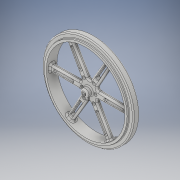
# Autodesk Inventor part: bepf_kolo_felga
Saved by Autodesk Inventor 2017 (Build 210142000, 142)
## iProperties
Created: 2016-11-22
Part Number: bepf_kolo_felga
Material: Tworzywo o ultrawysokiej masie cząsteczkowej, czarne
Document SubType Name: Modeling
Designer: gagato
Density: 0.94 g/cm^3
Appearance: Domyślna
Mass: 13.9753 g
Surface Area: 117.76 cm^2
Volume: 14.8674 cm^3
Author: gagato
Autodesk Inventor part; units mm, degrees
ref_plane "YZ Plane" through (0, 0, 0) normal (1, 0, 0) x (0, 1, 0)
ref_plane "XZ Plane" through (0, 0, 0) normal (0, 1, 0) x (-1, 0, 0)
ref_plane "XY Plane" through (0, 0, 0) normal (0, 0, 1) x (1, 0, 0)
sketch "Szkic1" plane through (0, 0, 0) normal (0, 0, 1) x (1, 0, 0)
  circle A0 centre (0, 0) radius 43.25
  dimension "d0" = 86.5
  constraints: 1 centre point, 1 coincident
  measures "d0" diameter of A0
extrude "Wyciągnięcie proste1" add sketch "Szkic1" along normal mid plane 10
sketch "Szkic2" plane through (0, 0, 5) normal (0, 0, 1) x (1, 0, 0)
  circle A0 centre (0, 0) radius 3.5
  circle A1 centre (0, 0) radius 37.25
  dimension "d3" = 7
  dimension "d4" = 74.5
  constraints: 2 centre point, 2 coincident
  measures "d3" diameter of A0
  measures "d4" diameter of A1
extrude "Wyciągnięcie proste2" cut sketch "Szkic2" against normal blind 3
sketch "Szkic3" plane through (0, 0, 5) normal (0, 0, 1) x (1, 0, 0)
  circle A0 centre (0, 0) radius 43.25 projected
  circle A1 centre (0, 0) radius 39.25
  dimension "d7" = 78.5
  constraints: 1 centre point, 1 coincident
  measures "d7" diameter of A1
extrude "Wyciągnięcie proste3" cut sketch "Szkic3" against normal blind 2
mirror "Odbij1" about plane through (0, 0, 0) normal (0, 0, 1) of "Wyciągnięcie proste2", "Wyciągnięcie proste3"
fillet "Zaokrąglenie1" radius 1 1 edges at (-43.25, 0, 3)
fillet "Zaokrąglenie2" radius 0.5 1 edges at (-39.25, 0, 3)
sketch "Szkic4" plane through (0, 0, 5) normal (0, 0, 1) x (1, 0, 0)
  circle A0 centre (0, 0) radius 3.5 projected
extrude "Wyciągnięcie proste4" add sketch "Szkic4" along normal blind 1.8
mirror "Odbij2" about plane through (0, 0, 0) normal (0, 0, 1) of "Zaokrąglenie2", "Zaokrąglenie1"
sketch "Szkic5" plane through (0, 0, -5) normal (0, 0, -1) x (-1, 0, 0)
  circle A0 centre (0, 0) radius 3.5 projected
extrude "Wyciągnięcie proste5" cut sketch "Szkic5" against normal up to surface (3 mm away)
sketch "Szkic7" plane through (0, 0, 2) normal (0, 0, 1) x (1, 0, 0)
  circle A0 centre (0, 0) radius 37.25 projected
  circle A1 centre (0, 0) radius 37.25 projected
  circle A2 centre (0, 0) radius 39.25 projected
  line L0 (-37.25, 0) -> (0, 0) construction
  circle A3 centre (0, 0) radius 3.5 construction
  circle A4 centre (-34.25, 0) radius 3 construction
  line L1 (-37.1323, 2.9582) -> (-0.0511, 3.4996) construction
  line L2 (-0.0511, -3.4996) -> (-37.1323, -2.9582) construction
  line L3 (-21.1281, -30.6784) -> (-3.0563, 1.7056) construction
  line L4 (3.0052, -1.7941) -> (-16.0043, -33.6367) construction
  line L5 (16.0043, -33.6367) -> (-3.0052, -1.7941) construction
  line L6 (3.0563, 1.7056) -> (21.1281, -30.6784) construction
  line L7 (37.1323, -2.9582) -> (0.0511, -3.4996) construction
  line L8 (0.0511, 3.4996) -> (37.1323, 2.9582) construction
  line L9 (21.1281, 30.6784) -> (3.0563, -1.7056) construction
  line L10 (-3.0052, 1.7941) -> (16.0043, 33.6367) construction
  line L11 (-16.0043, 33.6367) -> (3.0052, 1.7941) construction
  line L12 (-3.0563, -1.7056) -> (-21.1281, 30.6784) construction
  arc A5 (-9.2631, 3.3651) -> (-7.5458, 6.3395) centre (-9.2923, 5.3649) ccw
  line L13 (-7.5458, 6.3395) -> (-21.1281, 30.6784)
  line L14 (-9.2631, 3.3651) -> (-37.1323, 2.9582)
  arc A6 (-21.1281, 30.6784) -> (-37.1323, 2.9582) centre (0, 0) ccw
  arc A7 (-37.1323, -2.9582) -> (-21.1281, -30.6784) centre (0, 0) ccw
  arc A8 (-7.5458, -6.3395) -> (-9.2631, -3.3651) centre (-9.2923, -5.3649) ccw
  line L15 (-7.5458, -6.3395) -> (-21.1281, -30.6784)
  line L16 (-9.2631, -3.3651) -> (-37.1323, -2.9582)
  arc A9 (-16.0043, -33.6367) -> (16.0043, -33.6367) centre (0, 0) ccw
  arc A10 (1.7173, -9.7047) -> (-1.7173, -9.7047) centre (0, -10.7298) ccw
  line L17 (1.7173, -9.7047) -> (16.0043, -33.6367)
  line L18 (-1.7173, -9.7047) -> (-16.0043, -33.6367)
  arc A11 (21.1281, -30.6784) -> (37.1323, -2.9582) centre (0, 0) ccw
  arc A12 (9.2631, -3.3651) -> (7.5458, -6.3395) centre (9.2923, -5.3649) ccw
  line L19 (9.2631, -3.3651) -> (37.1323, -2.9582)
  line L20 (7.5458, -6.3395) -> (21.1281, -30.6784)
  arc A13 (37.1323, 2.9582) -> (21.1281, 30.6784) centre (0, 0) ccw
  arc A14 (7.5458, 6.3395) -> (9.2631, 3.3651) centre (9.2923, 5.3649) ccw
  line L21 (7.5458, 6.3395) -> (21.1281, 30.6784)
  line L22 (9.2631, 3.3651) -> (37.1323, 2.9582)
  arc A15 (16.0043, 33.6367) -> (-16.0043, 33.6367) centre (0, 0) ccw
  arc A16 (-1.7173, 9.7047) -> (1.7173, 9.7047) centre (0, 10.7298) ccw
  line L23 (-1.7173, 9.7047) -> (-16.0043, 33.6367)
  line L24 (1.7173, 9.7047) -> (16.0043, 33.6367)
  dimension "d33" = 7
  dimension "d34" = 6
  dimension "d37" = 360
  dimension "d39" = 4
  dimension "d42" = 360
  constraints: 50 end point, 32 point on circle, 14 centre point, 7 tangent, 3 point on line, 2 coincident, 2 collinear, 1 horizontal, 98 other
  measures "d33" diameter of A3
  measures "d34" diameter of A4
  measures "d39" diameter of A5
extrude "Wyciągnięcie proste6" cut sketch "Szkic7" against normal through all contours L22 A14 L21 A0 | A0 L20 A12 L19 | L24 A16 L23 A0 | A0 L18 A10 L17 | L13 A5 L14 A0 | A0 L16 A8 L15
sketch "Szkic8" plane through (0, 0, 2) normal (0, 0, 1) x (1, 0, 0)
  line L0 (-6.35, 0) -> (6.35, 0) construction
  line L1 (0, 0) -> (-4.7625, 8.22) construction
  line L2 (0, 0) -> (-9.5, -0.0144) construction
  line L3 (0, 0) -> (-4.7375, -8.2345) construction
  line L4 (0, 0) -> (4.7625, -8.22) construction
  line L5 (0, 0) -> (9.5, 0.0144) construction
  line L6 (0, 0) -> (4.7375, 8.2345) construction
  point P0 (-4.7625, 8.25)
  dimension "d51" = 12.7
  dimension "d63" = 9.5
  dimension "d66" = 360
  constraints: 14 end point, 9 coincident, 1 horizontal, 1 midpoint, 23 other
  measures "d51" distance of L0.start L0.end
  measures "d63" distance of L1.start L1.end
hole "Otwór1" at (6.35, 0, 2) at (-4.7625, 8.25, 2) at (-6.35, 0, 2) at (4.7625, -8.22, 2) at (-4.7375, -8.2345, 2) at (4.7375, 8.2345, 2) direction (0, 0, -1) diameter 3 end through all
sketch "Szkic9" plane through (0, 0, 2) normal (0, 0, 1) x (1, 0, 0)
  arc A0 (-1.5811, 0.75) -> (1.5811, 0.75) centre (0, 0) ccw
  arc A1 (1.7173, -9.7047) -> (-1.7173, -9.7047) centre (0, -10.7298) ccw construction
  circle A2 centre (0, 0) radius 0.75 construction
  line L0 (1.5811, 0.75) -> (-1.5811, 0.75)
  line L1 (0.75, 0.75) -> (0.75, -10.7298) construction
  line L2 (0.75, -10.7298) -> (0, -10.7298) construction
  line L3 (0, -10.7298) -> (-0.75, -10.7298) construction
  line L4 (-0.75, -10.7298) -> (-0.75, 0.75) construction
  line L5 (-0.75, -1.5811) -> (-0.75, -10.7298)
  line L6 (0.75, -10.7298) -> (0.75, -1.5811)
  line L7 (-0.75, -10.7298) -> (0.75, -10.7298)
  dimension "d59" = 3.5
  dimension "d60" = 1.5
  constraints: 16 end point, 5 point on line, 4 point on circle, 3 perpendicular, 3 tangent, 2 centre point, 2 coincident, 2 collinear, 1 horizontal
  measures "d59" diameter of A0
  measures "d60" diameter of A2
extrude "Wyciągnięcie proste7" cut sketch "Szkic9" along normal through all both and the other way through all
fillet "Zaokrąglenie5" radius 1.5 38 edges at (7.5603, -4.3649, 2) (23.1977, -3.1617, 2) (14.337, -18.509, 2) (0, 8.7298, -2) (-8.8608, 21.6707, -2) (8.8608, 21.6707, -2) (0, 8.7298, 2) (8.8608, 21.6707, 2) (-8.8608, 21.6707, 2) (7.5603, -4.3649, -2) (14.337, -18.509, -2) (23.1977, -3.1617, -2) (7.5603, 4.3649, -2) (23.1977, 3.1617, -2) (14.337, 18.509, -2) (-7.5603, -4.3649, 2) (-14.337, -18.509, 2) (-23.1977, -3.1617, 2) (-7.5603, 4.3649, 2) (-14.337, 18.509, 2) (-23.1977, 3.1617, 2) (1.3014, -9.2112, 2) (-1.3014, -9.2112, 2) (8.8608, -21.6707, 2) (-8.8608, -21.6707, 2) (-1.3014, -9.2112, -2) (1.3014, -9.2112, -2) (8.8608, -21.6707, -2) (-8.8608, -21.6707, -2) (-7.5603, -4.3649, -2) (-14.337, -18.509, -2) (-23.1977, -3.1617, -2) (-7.5603, 4.3649, -2) (-23.1977, 3.1617, -2) (-14.337, 18.509, -2) (14.337, 18.509, 2) (23.1977, 3.1617, 2) (7.5603, 4.3649, 2)
fillet "Zaokrąglenie3" radius 1.5 2 edges at (2.7272, -2.1937, 6.8) (-2.1937, 2.7272, 6.8) curvature continuous yes
fillet "Zaokrąglenie4" radius 1 2 edges at (2.7272, -2.1937, 2) (-2.1937, 2.7272, 2)
fillet "Zaokrąglenie7" radius 1.5 50 edges at (-37.25, 0, 2) (-37.1602, -2.5846, 1.4901) (-37.1323, -2.9582, 0) (-37.16, -2.5872, -1.4872) (-37.25, 0, -2) (-37.16, 2.5872, -1.4872) (-37.1323, 2.9582, 0) (-37.16, 2.5885, 1.4856) (16.3395, 33.4751, -1.4872) (18.625, 32.2594, -2) (20.8206, 30.888, -1.4872) (21.1281, 30.6784, 0) (20.8188, 30.8891, 1.4896) (18.625, 32.2594, 2) (16.3418, 33.474, 1.4901) (16.0043, 33.6367, 0) (-16.3414, 33.4742, 1.4896) (-16.0043, 33.6367, 0) (-16.3395, 33.4751, -1.4872) (-18.625, 32.2594, -2) (-20.8206, 30.888, -1.4872) (-21.1281, 30.6784, 0) (-20.8188, 30.8891, 1.4896) (-18.625, 32.2594, 2) (-20.8188, -30.8891, 1.4896) (-21.1281, -30.6784, 0) (-20.8206, -30.888, -1.4872) (-18.625, -32.2594, -2) (-16.3395, -33.4751, -1.4872) (-16.0043, -33.6367, 0) (-16.3382, -33.4757, 1.4856) (-18.625, -32.2594, 2) (16.3414, -33.4742, 1.4896) (16.0043, -33.6367, 0) (16.3395, -33.4751, -1.4872) (18.625, -32.2594, -2) (20.8206, -30.888, -1.4872) (21.1281, -30.6784, 0) (20.8217, -30.8872, 1.4856) (18.625, -32.2594, 2) (37.1602, -2.5846, 1.4901) (37.1323, -2.9582, 0) (37.16, -2.5872, -1.4872) (37.2429, 0.7285, -2) (37.2429, -0.7285, -2) (37.16, 2.5872, -1.4872) (37.1323, 2.9582, 0) (37.16, 2.5885, 1.4856) (37.2429, -0.7285, 2) (37.2429, 0.7285, 2)
sketch "Szkic10" plane through (0, 0, 0) normal (0, 0, 1) x (1, 0, 0)
  line L0 (0, 0) -> (-7.9992, 13.8569) construction
  circle A0 centre (-4.7625, 8.25) radius 1.5 construction
  line L1 (0, 0) -> (-15.9984, 27.7137) construction
  arc A1 (-15.0957, 28.25) -> (-16.9142, 27.2002) centre (-15.9984, 27.7137) ccw
  arc A2 (-9.0895, 13.2455) -> (-6.9245, 14.4953) centre (-7.9992, 13.8569) ccw
  line L2 (-6.9245, 14.4953) -> (-15.0957, 28.25)
  line L3 (-16.9142, 27.2002) -> (-9.0895, 13.2455)
  dimension "d68" = 16
  dimension "d69" = 32
  dimension "d70" = 2.1
  dimension "d71" = 2.5
  constraints: 8 end point, 4 point on circle, 4 tangent, 2 centre point, 2 coincident, 2 point on line
  measures "d68" distance of L0.start L0.end
  measures "d69" distance of L0.start L1.end
  measures "d70" diameter of A1
  measures "d71" diameter of A2
extrude "Wyciągnięcie proste8" cut sketch "Szkic10" along normal through all both and the other way through all
pattern_circular "Szyk kołowy1" count 6 over 360 about axis through (0, 0, -5) along (0, 0, -1) of "Wyciągnięcie proste8"
fillet "Zaokrąglenie8" radius 0.5 48 edges at (-7.3743, 12.7743, 2) (-13.0019, 20.2229, 2) (-16.5233, 28.6231, 2) (-11.0101, 21.3727, 2) (-16.5233, 28.6231, -2) (-13.0019, 20.2229, -2) (-7.3743, 12.7743, -2) (-11.0101, 21.3727, -2) (16.5267, 28.6212, 2) (13.0042, 20.2213, 2) (7.3757, 12.7734, 2) (11.0126, 21.3714, 2) (16.5267, 28.6212, -2) (11.0126, 21.3714, -2) (7.3757, 12.7734, -2) (13.0042, 20.2213, -2) (33.05, -0.0019, 2) (24.0143, -1.1513, 2) (14.75, -0.0009, 2) (24.0144, 1.1485, 2) (33.05, -0.0019, -2) (24.0144, 1.1485, -2) (14.75, -0.0009, -2) (24.0143, -1.1513, -2) (7.3743, -12.7743, -2) (11.0101, -21.3727, -2) (16.5233, -28.6231, -2) (13.0019, -20.2229, -2) (7.3743, -12.7743, 2) (13.0019, -20.2229, 2) (16.5233, -28.6231, 2) (11.0101, -21.3727, 2) (-16.5267, -28.6212, -2) (-11.0126, -21.3714, -2) (-7.3757, -12.7734, -2) (-13.0042, -20.2213, -2) (-16.5267, -28.6212, 2) (-13.0042, -20.2213, 2) (-7.3757, -12.7734, 2) (-11.0126, -21.3714, 2) (-33.05, 0.0019, -2) (-24.0144, -1.1485, -2) (-14.75, 0.0009, -2) (-24.0143, 1.1513, -2) (-33.05, 0.0019, 2) (-24.0143, 1.1513, 2) (-14.75, 0.0009, 2) (-24.0144, -1.1485, 2)
